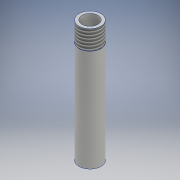
# Autodesk Inventor part: Connecting Rod
Saved by Autodesk Inventor 2017 (Build 210142000, 142)
## iProperties
Created: 2020-05-28
Part Number: Connecting Rod
Material: Aluminum 6061
Document SubType Name: Modeling
Designer: Sid
Density: 2.7 g/cm^3
Appearance: Aluminum - Flat
Mass: 32.7228 g
Surface Area: 99.7638 cm^2
Volume: 12.1196 cm^3
Author: Sid
Autodesk Inventor part; units mm, degrees
ref_plane "YZ Plane" through (0, 0, 0) normal (1, 0, 0) x (0, 1, 0)
ref_plane "XZ Plane" through (0, 0, 0) normal (0, 1, 0) x (-1, 0, 0)
ref_plane "XY Plane" through (0, 0, 0) normal (0, 0, 1) x (1, 0, 0)
sketch "Sketch1" plane through (0, 0, 0) normal (0, 0, 1) x (1, 0, 0)
  circle A0 centre (0, 0) radius 9
  circle A1 centre (0, 0) radius 6.5
  dimension "d0" = 18
  dimension "d1" = 13
  constraints: 2 centre point, 2 coincident
  measures "d0" diameter of A0
  measures "d1" diameter of A1
extrude "Extrusion1" add sketch "Sketch1" along normal blind 100
sketch "Sketch2" plane through (0, 0, 100) normal (0, 0, 1) x (1, 0, 0)
  circle A0 centre (0, 0) radius 8.94
  circle A1 centre (0, 0) radius 12.634
  dimension "d4" = 17.88
  constraints: 2 centre point, 2 coincident
  measures "d4" diameter of A0
extrude "Extrusion2" cut sketch "Sketch2" against normal blind 16
thread "Thread1" size "M18x2.5" class "6g" standard "ANSI Metric M Profile" full length
body "Solid1"
